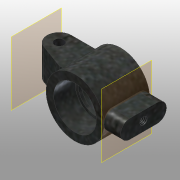
# Autodesk Inventor part: 500-007
Saved by Autodesk Inventor 2016 (Build 200138000, 138)
## iProperties
Created: 2015-04-18
Part Number: 500-007
Material: Steel
Document SubType Name: Modeling
Designer: Station9
Density: 7.85 g/cm^3
Appearance: Plate
Mass: 25.6143 g
Surface Area: 26.1117 cm^2
Volume: 3.26297 cm^3
Author: Station9
Autodesk Inventor part; units mm, degrees
ref_plane "XZ Plane" through (0, 0, 0) normal (0, 1, 0) x (-1, 0, 0)
ref_plane "XY Plane" through (0, 0, 0) normal (0, 0, 1) x (1, 0, 0)
sketch "Sketch1" plane through (0, 0, 0) normal (0, 1, 0) x (-1, 0, 0)
  circle A0 centre (0, 0) radius 9.5
  dimension "d0" = 19
  constraints: 1 centre point, 1 coincident
  measures "d0" diameter of A0
extrude "Extrusion1" add sketch "Sketch1" along normal blind 15
sketch "Sketch2" plane through (0, 0, 0) normal (0, -1, 0) x (1, 0, 0)
  circle A0 centre (0, 0) radius 9.5 projected
  circle A1 centre (0, 0) radius 7
  dimension "d3" = 14
  constraints: 1 centre point, 1 coincident
  measures "d3" diameter of A1
extrude "Extrusion2" cut sketch "Sketch2" against normal blind 7 contours A1
sketch "Sketch3" plane through (0, 15, 0) normal (0, 1, 0) x (1, 0, 0)
  circle A0 centre (0, 0) radius 9.5 projected
  circle A1 centre (0, 0) radius 7
  dimension "d6" = 14
  constraints: 1 centre point, 1 coincident
  measures "d6" diameter of A1
extrude "Extrusion3" cut sketch "Sketch3" against normal blind 7 contours A1
sketch "Sketch5" plane through (0, 7, 0) normal (0, -1, 0) x (1, 0, 0)
  circle A0 centre (0, 0) radius 7 projected
  circle A1 centre (0, 0) radius 6
  dimension "d9" = 12
  constraints: 1 centre point, 1 coincident
  measures "d9" diameter of A1
extrude "Extrusion4" cut sketch "Sketch5" against normal through all contours A1
ref_plane "Work Plane1" through (9.5, 0, 0) normal (1, 0, 0) x (0, 1, 0)
sketch "Sketch6" plane through (9.5, 0, 0) normal (1, 0, 0) x (0, 1, 0)
  line L0 (0, 9.5) -> (15, 9.5) projected
  line L1 (12, 0) -> (3, 0) construction
  line L2 (7, -7) -> (7, 7) projected
  line L3 (12, 3) -> (3, 3)
  line L4 (3, -3) -> (12, -3)
  arc A0 (12, -3) -> (12, 3) centre (12, 0) ccw
  arc A1 (3, 3) -> (3, -3) centre (3, 0) ccw
  line L5 (0, 9.5) -> (0, -9.5) projected
  line L6 (15, -9.5) -> (15, 9.5) projected
  point P0 (0, 0)
  point P1 (7.5, 0)
  point P2 (15, 0)
  dimension "d13" = 3
  constraints: 8 end point, 6 tangent, 4 point on circle, 2 centre point, 2 midpoint, 1 horizontal alignment, 1 parallel, 1 perpendicular
  measures "d13" radius of A1
extrude "Extrusion5" add sketch "Sketch6" along normal blind 5.5 and the other way blind 1.25 contours A1 L3 L2 L4 | A0 L4 L2 L3
sketch "Sketch7" plane through (0, 0, 0) normal (0, 0, 1) x (1, 0, 0)
  line L0 (-7, 7) -> (-7, 0) construction
  line L1 (-7, 0) -> (-9.5, 0) construction
  line L2 (-9.5, 0) -> (-9.5, 15) construction
  line L3 (-9.5, 15) -> (-7, 15) construction
  line L4 (-7, 15) -> (-7, 8) construction
  line L5 (-7, 8) -> (-6, 8) construction
  line L6 (-6, 8) -> (-6, 7) construction
  line L7 (-6, 7) -> (-7, 7) construction
  line L8 (7, 0) -> (7, 7) construction
  line L9 (7, 7) -> (6, 7) construction
  line L10 (6, 7) -> (6, 8) construction
  line L11 (6, 8) -> (7, 8) construction
  line L12 (7, 8) -> (7, 15) construction
  line L13 (7, 15) -> (9.5, 15) construction
  line L14 (9.5, 15) -> (15, 15) construction
  line L15 (15, 15) -> (15, 0) construction
  line L16 (15, 0) -> (9.5, 0) construction
  line L17 (9.5, 0) -> (7, 0) construction
  line L18 (-9.5, 15) -> (-16.15, 15)
  line L19 (-17.5181, 7.2412) -> (-9.5, 4.3229)
  line L20 (-9.5, 4.3229) -> (-7.9897, 4.3229)
  line L21 (-7.9897, 4.3229) -> (-7.9897, 15)
  line L22 (-9.5, 15) -> (-7.9897, 15)
  line L23 (9.5, 15) -> (-9.5, 15) projected
  arc A0 (-16.15, 15) -> (-17.5181, 7.2412) centre (-16.15, 11) ccw
  point P0 (0, 0)
  dimension "d18" = 4
  dimension "d19" = 20
  dimension "d21" = 16.15
  constraints: 10 end point, 2 horizontal, 2 point on circle, 2 point on line, 2 tangent, 1 centre point, 1 collinear, 1 vertical
  measures "d18" radius of A0
  measures "d19" angle of L18 L19
  measures "d21" horizontal distance of A0.centre point (0, 0)
extrude "Extrusion6" add sketch "Sketch7" along normal mid plane 10
hole "Hole1" at (-16.15, 11, 5) direction (0, 0, -1) diameter 3.1 end through all
sketch "Sketch8" plane through (15, 0, 0) normal (1, 0, 0) x (0, 0, -1)
  arc A0 (3, 12) -> (-3, 12) centre (0, 12) ccw projected
  line L0 (0, 15) -> (0, 7.5)
  point P0 (0, 0)
  constraints: 2 end point, 1 point on circle, 1 vertical
hole "Hole2" at (15, 7.5, 0) direction (-1, 0, 0) diameter 2.459 depth 6 tip angle 118 thread size "M3x0.5" class "6H" standard "ISO Metric profile"
ref_plane "Work Plane2" through (-20.15, 11, 0) normal (1, 0, 0) x (0, 1, 0)
sketch "Sketch9" plane through (-20.15, 11, 0) normal (1, 0, 0) x (0, 1, 0)
  line L0 (-1.55, 5) -> (1.55, 5) projected
  line L1 (0, 5) -> (0, 0)
  point P0 (-11, 0)
  constraints: 2 end point, 1 midpoint, 1 vertical
hole "Hole3" at (-20.15, 11, 0) direction (1, 0, 0) diameter 2.459 depth 4 tip angle 118 thread size "M3x0.5" class "6H" standard "ISO Metric profile"
body "Solid1"
